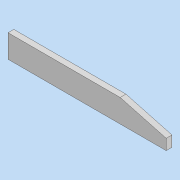
# Autodesk Inventor part: bodySidePlate
Saved by Autodesk Inventor 2021 (Build 250183000, 183)
## iProperties
Created: 2021-02-01
Part Number: bodySidePlate
Material: Generic
Document SubType Name: Modeling
Designer: garre
Density: 1 g/cm^3
Appearance: Default
Author: garre
Autodesk Inventor part; units mm, degrees
ref_plane "YZ Plane" through (0, 0, 0) normal (1, 0, 0) x (0, 1, 0)
ref_plane "XZ Plane" through (0, 0, 0) normal (0, 1, 0) x (-1, 0, 0)
ref_plane "XY Plane" through (0, 0, 0) normal (0, 0, 1) x (1, 0, 0)
sketch "Sketch1" plane through (0, 0, 0) normal (0, 0, 1) x (1, 0, 0)
  line L0 (0, 0) -> (495.3, 0)
  line L1 (495.3, 0) -> (495.3, 101.6)
  line L2 (495.3, 101.6) -> (0, 101.6)
  line L3 (0, 101.6) -> (0, 0)
  line L4 (495.3, 101.6) -> (698.5, 101.6)
  line L5 (698.5, 101.6) -> (698.5, 0)
  line L6 (698.5, 0) -> (495.3, 0)
  line L7 (495.3, 0) -> (495.3, 101.6)
  line L8 (495.3, 101.6) -> (698.5, 47.1527)
  dimension "d0" = 495.3
  dimension "d1" = 101.6
  dimension "d2" = 203.2
  dimension "d4" = 15
  constraints: 18 end point, 5 parallel, 2 horizontal, 2 perpendicular, 1 point on line
  measures "d0" distance of L1.end L2.end
  measures "d1" distance of L2.end L0.start
  measures "d2" distance of L1.end L4.end
  measures "d4" angle of L4 L8
extrude "Extrusion1" add sketch "Sketch1" along normal blind 25.4 contours L3 L2 L1 L0 | L1 L8 L5 L6
equation "\"d0\" = bodyLengthUntilNut"
equation "\"d1\" = bodyHeight"
equation "\"d2\" = extensionLength"
equation "\"d4\" = postNutAngle"
equation "\"d5\" = woodThickness"
equation "\"bodyLengthUntilNut\" = 495.3"
equation "\"postNutAngle\" = 15deg"
equation "\"woodThickness\" = 25.4"
equation "\"slantLength\" = 127"
equation "\"extensionLength\" = 203.2"
equation "\"bodyHeight\" = 101.6"
body "Solid1"
